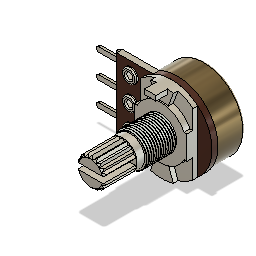
POT10K (Autodesk Fusion 360 design; units mm, degrees)
Autodesk Fusion 360 part; units mm, degrees
sketch "Sketch1" plane through (0, 0, 0) normal (0, 0, 1) x (1, 0, 0)
  circle A0 centre (0, 0) radius 8.2
  dimension "d1" = 16.4
  constraint coincident A0.centre origin
  measures "d1" diameter of A0
extrude "Extrude1" add sketch "Sketch1" along normal blind 6
sketch "Sketch2" plane through (0, 0, 6) normal (0, 0, 1) x (1, 0, 0)
  circle A0 centre (0, 0) radius 8.2
  line L0 (0, 0) -> (-11.5, 0)
  line L1 (-11.5, 0) -> (-11.5, 7.6)
  line L2 (-11.5, 7.6) -> (-3.8066, 7.6)
  line L3 (-11.5, 0) -> (-11.5, -7.6)
  line L4 (-11.5, -7.6) -> (-3.8066, -7.6)
  arc A1 (-3.8066, -7.6) -> (-3.8066, 7.6) centre (0, 0) ccw
  dimension "d4" = 17
  dimension "d5" = 11.5
  dimension "d6" = 7.6
  dimension "d7" = 7.6
  constraint concentric A0 A1
  constraint coincident A0.centre L0.start
  constraint horizontal L0
  constraint perpendicular L0 L1
  constraint perpendicular L1 L2
  constraint perpendicular L0 L3
  constraint perpendicular L3 L4
  measures "d4" diameter of A1
  measures "d5" distance of A0.centre L0.end
  measures "d6" distance of L0.end L1.end
  measures "d7" distance of L0.end L3.end
extrude "Extrude2" add sketch "Sketch2" along normal blind 1.25 contours A0 | L1 L2 L3 L4 A1
fillet "Fillet1" radius 0.5 1 edges at (-7.6451, -2.9652, 0)
sketch "Sketch3" plane through (0, 0, 7.25) normal (0, 0, 1) x (1, 0, 0)
  line L0 (-11.5, 7.6) -> (-11.5, -7.6)
  line L1 (-11.5, -7.6) -> (-3.8066, -7.6)
  arc A0 (-3.8066, -7.6) -> (-3.8066, 7.6) centre (0, 0) ccw
  line L2 (-3.8066, 7.6) -> (-11.5, 7.6)
  circle A1 centre (0, 0) radius 8.5
  line L3 (-5.5, 0) -> (-5.5, 6.4807)
  line L4 (5.5, 6.4807) -> (5.5, -6.4807)
  line L5 (-5.5, -6.4807) -> (-5.5, 0)
  circle A2 centre (0, 0) radius 8.495
  dimension "d15" = 16.99
  constraint concentric A0 A1
  constraint vertical L3
  constraint coincident A1 L3.end
  constraint coincident A0 L4.start
  constraint coincident A1 L5.start
  constraint coincident A0 L4.end
  constraint concentric A1 A2
  measures "d15" diameter of A2
extrude "Extrude3" add sketch "Sketch3" along normal blind 1 contours A0 A1 L3 L4 A2 | A0 A1 L4 L5 A2 | L3 L4 L5 A2
sketch "Sketch4" plane through (0, 0, 8.25) normal (0, 0, 1) x (1, 0, 0)
  arc A0 (-5.5, -6.4742) -> (5.5, -6.4742) centre (0, 0) ccw
  line L0 (5.5, -6.4742) -> (5.5, 6.4742)
  arc A1 (5.5, 6.4742) -> (-5.5, 6.4742) centre (0, 0) ccw
  line L1 (-5.5, 6.4742) -> (-5.5, -6.4742)
  line L2 (5.5, 0) -> (5.5, 2.5)
  line L3 (-5.5, 2.5) -> (-5.5, -2.5)
  line L4 (5.5, -2.5) -> (5.5, 0)
  line L5 (-5.5, -2.5) -> (-4.899, -2.5)
  line L6 (4.899, -2.5) -> (5.5, -2.5)
  arc A2 (-4.899, -2.5) -> (4.899, -2.5) centre (0, 0) ccw
  arc A3 (4.899, 2.5) -> (-4.899, 2.5) centre (0, 0) ccw
  line L7 (5.5, 2.5) -> (4.899, 2.5)
  line L8 (-4.899, 2.5) -> (-5.5, 2.5)
  dimension "d18" = 2.5
  dimension "d19" = 5
  constraint coincident A0.centre A1.centre
  constraint tangent L0 A2
  constraint midpoint L0 L2.start
  constraint parallel L0 L2
  constraint coincident L1 L3.start
  constraint perpendicular L1 L7
  constraint perpendicular L3 L7
  constraint coincident L0 L4.start
  constraint perpendicular L0 L5
  constraint coincident A3.end L7
  constraint collinear L5 L6
  constraint concentric A2 A3
  constraint collinear L7 L8
  measures "d18" distance of L2.start L2.end
  measures "d19" distance of L3.start L3.end
extrude "Extrude4" add sketch "Sketch4" along normal blind 1.25 contours L0 L1 L2 L3 L4 L5 L6 A2 A3 L7 L8
sketch "Sketch5" plane through (0, 0, 8.25) normal (0, 0, 1) x (1, 0, 0)
  line L0 (5.5, -2.5) -> (4.899, -2.5)
  arc A0 (-4.899, -2.5) -> (4.899, -2.5) centre (0, 0) ccw
  line L1 (-4.899, -2.5) -> (-5.5, -2.5)
  line L2 (-5.5, -2.5) -> (-5.5, -6.4742)
  arc A1 (-5.5, -6.4742) -> (5.5, -6.4742) centre (0, 0) ccw
  line L3 (5.5, -6.4742) -> (5.5, -2.5)
  circle A2 centre (0, 0) radius 8.495
  line L4 (0, 0) -> (1.35, 0)
  line L5 (1.35, 0) -> (1.35, 0.0007)
  circle A3 centre (0, 0) radius 5.5
  line L6 (-1.35, 5.3317) -> (-2.4, 8.1489)
  line L7 (1.35, 5.3317) -> (2.4, 8.1489)
  line L8 (1.35, -5.3317) -> (2.4, -8.1489)
  line L9 (-2.3914, -8.1514) -> (-1.35, -5.3317)
  dimension "d23" = 1.35
  dimension "d26" = 11
  constraint coincident A0.centre A1.centre
  constraint horizontal L4
  constraint coincident A2 L7.end
  constraint coincident A2 L6.end
  constraint coincident A1 L9.start
  constraint coincident A2 L9.start
  constraint coincident A1 L8.end
  constraint coincident A3 L6.start
  constraint coincident A3 L7.start
  constraint coincident A3 L8.start
  constraint coincident A3 L9.end
  measures "d23" distance of A0.centre L5.end
  measures "d26" diameter of A3
extrude "Extrude5" add sketch "Sketch5" along normal blind 1 contours A0 A1 A2 A3 L8 L9 | A2 A3 L6 L7
sketch "Sketch6" plane through (0, 0, 9.25) normal (0, 0, 1) x (1, 0, 0)
  arc A0 (1.35, 5.3317) -> (-1.35, 5.3317) centre (0, 0) ccw
  line L0 (1.35, 5.3317) -> (2.4, 8.1489)
  arc A1 (2.4, 8.1489) -> (-2.4, 8.1489) centre (0, 0) ccw
  line L1 (-2.4, 8.1489) -> (-1.35, 5.3317)
  circle A2 centre (0, 0) radius 7.5
  line L2 (0, 0) -> (1.2, 0)
  line L3 (1.2, 0) -> (1.2, 9)
  line L4 (1.2, 9) -> (-1.2, 9)
  line L5 (-1.2, 9) -> (-1.2, 6.8335)
  dimension "d29" = 15
  dimension "d30" = 1.2
  dimension "d31" = 2.4
  constraint concentric A0 A2
  constraint coincident A0.centre A1.centre
  constraint horizontal L2
  constraint perpendicular L2 L3
  constraint perpendicular L3 L4
  constraint perpendicular L4 L5
  measures "d29" diameter of A2
  measures "d30" distance of A0.centre L2.end
  measures "d31" distance of L3.end L4.end
extrude "Extrude6" add sketch "Sketch6" along normal blind 2.5 contours A1 A2 L3 L5
sketch "Sketch7" plane through (0, 0, 9.5) normal (0, 0, 1) x (1, 0, 0)
  line L0 (-4.899, 2.5) -> (-5.5, 2.5)
  line L1 (-5.5, 2.5) -> (-5.5, -2.5)
  line L2 (-5.5, -2.5) -> (-4.899, -2.5)
  arc A0 (-4.899, -2.5) -> (4.899, -2.5) centre (0, 0) ccw
  line L3 (4.899, -2.5) -> (5.5, -2.5)
  line L4 (5.5, -2.5) -> (5.5, 2.5)
  line L5 (5.5, 2.5) -> (4.899, 2.5)
  arc A1 (4.899, 2.5) -> (-4.899, 2.5) centre (0, 0) ccw
  circle A2 centre (0, 0) radius 3.5
  dimension "d34" = 7
  constraint coincident A0.centre A1.centre
  measures "d34" diameter of A2
extrude "Extrude7" add sketch "Sketch7" along normal blind 6.4 contours A2
thread "Thread1" "ISO Metric profile 7.0 M7x0.5 6g" major diameter 6.927 minor diameter 6.3505 pitch 0.5 angle 60 modelled right hand crest width 0.0685 on face at (3.4547, -0.5614, 13.7667) crest through (3.4635, 0, 9.375)
sketch "Sketch8" plane through (0, 0, 15.9) normal (0, 0, 1) x (1, 0, 0)
  spline S0 degree 3 poles (-1.8886, -2.5525) (-1.5648, -2.8146) (-1.1927, -3.0103) (-0.3879, -3.2513) (0.0378, -3.2917) (0.8877, -3.2078) (1.3036, -3.0816) (2.0704, -2.6747) (2.4127, -2.3957) (2.8876, -1.8243) (3.0502, -1.5642) (3.3033, -1.0046) (3.392, -0.7075) (3.44, -0.4025) knots 0 0 0 0 0.124949 0.124949 0.251948 0.251948 0.380996 0.380996 0.512093 0.512093 0.60358 0.60358 0.696049 0.696049 0.696049 0.696049
  arc A0 (3.44, -0.4025) -> (2.5464, 2.3476) centre (0, 0) ccw
  spline S1 degree 3 poles (2.5464, 2.3476) (2.2304, 2.6642) (1.8561, 2.9164) (1.0377, 3.2593) (0.6025, 3.3492) (-0.2709, 3.3556) (-0.7006, 3.2748) (-1.4981, 2.9543) (-1.8591, 2.7203) (-2.3721, 2.2213) (-2.5516, 1.9927) (-2.8429, 1.4963) (-2.9541, 1.2313) (-3.0282, 0.955) knots 0 0 0 0 0.134177 0.134177 0.266302 0.266302 0.396376 0.396376 0.524397 0.524397 0.611348 0.611348 0.697316 0.697316 0.697316 0.697316
  arc A1 (-3.0282, 0.955) -> (-1.8886, -2.5525) centre (0, 0) ccw
  circle A2 centre (0, 0) radius 3.05
  dimension "d37" = 6.1
  constraint concentric A0 A2
  measures "d37" diameter of A2
extrude "Extrude8" add sketch "Sketch8" along normal blind 8.3 contours A2
chamfer "Chamfer1" distance 0.5 angle 45 1 edges at (-2.8436, -1.1029, 24.2)
sketch "Sketch9" plane through (0, 0, 24.2) normal (0, 0, 1) x (1, 0, 0)
  circle A0 centre (0, 0) radius 2.55
  circle A1 centre (0, 0) radius 3.05
  circle A2 centre (0, 0) radius 2.55
  line L0 (0, 0) -> (0, 3.05)
  line L1 (0, 0) -> (1.1557, 3.557)
  line L2 (0, 0) -> (0.3989, 2.5186)
  line L3 (0, 0) -> (2.55, 0) construction
  line L4 (0, 3.05) -> (0.3989, 2.5186)
  line L5 (0.9425, 2.9007) -> (0.3989, 2.5186)
  line L6 (0, 3.05) -> (-0.3989, 2.5186)
  line L7 (-0.9425, 2.9007) -> (-0.3989, 2.5186)
  line L8 (-0.9425, 2.9007) -> (-1.1577, 2.2721)
  line L9 (-1.7927, 2.4675) -> (-1.1577, 2.2721)
  line L10 (-1.7927, 2.4675) -> (-1.8031, 1.8031)
  line L11 (-2.4675, 1.7927) -> (-1.8031, 1.8031)
  line L12 (-2.4675, 1.7927) -> (-2.2721, 1.1577)
  line L13 (-2.9007, 0.9425) -> (-2.2721, 1.1577)
  line L14 (-2.9007, 0.9425) -> (-2.5186, 0.3989)
  line L15 (-3.05, 0) -> (-2.5186, 0.3989)
  line L16 (-3.05, 0) -> (-2.5186, -0.3989)
  line L17 (-2.9007, -0.9425) -> (-2.5186, -0.3989)
  line L18 (-2.9007, -0.9425) -> (-2.2721, -1.1577)
  line L19 (-2.4675, -1.7927) -> (-2.2721, -1.1577)
  line L20 (-2.4675, -1.7927) -> (-1.8031, -1.8031)
  line L21 (-1.7927, -2.4675) -> (-1.8031, -1.8031)
  line L22 (-1.7927, -2.4675) -> (-1.1577, -2.2721)
  line L23 (-0.9425, -2.9007) -> (-1.1577, -2.2721)
  line L24 (-0.9425, -2.9007) -> (-0.3989, -2.5186)
  line L25 (0, -3.05) -> (-0.3989, -2.5186)
  line L26 (0, -3.05) -> (0.3989, -2.5186)
  line L27 (0.9425, -2.9007) -> (0.3989, -2.5186)
  line L28 (0.9425, -2.9007) -> (1.1577, -2.2721)
  line L29 (1.7927, -2.4675) -> (1.1577, -2.2721)
  line L30 (1.7927, -2.4675) -> (1.8031, -1.8031)
  line L31 (2.4675, -1.7927) -> (1.8031, -1.8031)
  line L32 (2.4675, -1.7927) -> (2.2721, -1.1577)
  line L33 (2.9007, -0.9425) -> (2.2721, -1.1577)
  line L34 (2.9007, -0.9425) -> (2.5186, -0.3989)
  line L35 (3.05, 0) -> (2.5186, -0.3989)
  line L36 (3.05, 0) -> (2.5186, 0.3989)
  line L37 (2.9007, 0.9425) -> (2.5186, 0.3989)
  line L38 (2.9007, 0.9425) -> (2.2721, 1.1577)
  line L39 (2.4675, 1.7927) -> (2.2721, 1.1577)
  line L40 (2.4675, 1.7927) -> (1.8031, 1.8031)
  line L41 (1.7927, 2.4675) -> (1.8031, 1.8031)
  line L42 (1.7927, 2.4675) -> (1.1577, 2.2721)
  line L43 (0.9425, 2.9007) -> (1.1577, 2.2721)
  dimension "d41" = 6.1
  dimension "d42" = 162
  dimension "d43" = 81
  dimension "d45" = 360
  constraint concentric A0 A1
  constraint concentric A1 A2
  constraint coincident A0.centre A1.centre
  constraint coincident A1 L0.end
  constraint vertical L0
  constraint horizontal L3
  constraint coincident A2 L2.end
  constraint coincident L1 L5.start
  constraint coincident A1 L5.start
  measures "d41" diameter of A1
  measures "d42" angle of L0 L1
  measures "d43" angle of L2 L3
extrude "Extrude9" cut sketch "Sketch9" against normal blind 6.7 contours A1 L36 L37 | A1 L34 L35 | A1 L38 L39 | A1 L32 L33 | A1 L40 L41 | A1 L30 L31 | A1 L42 L43 | A1 L28 L29 | A1 L4 L5 | A1 L26 L27 | A1 L6 L7 | A1 L24 L25 | A1 L8 L9 | A1 L22 L23 | A1 L10 L11 | A1 L20 L21 | A1 L12 L13 | A1 L18 L19 | A1 L14 L15 | A1 L16 L17
sketch "Sketch10" plane through (0, 0, 24.2) normal (0, 0, 1) x (1, 0, 0)
  arc A0 (-2.5186, 0.3989) -> (-2.5186, -0.3989) centre (0, 0) ccw
  arc A1 (-2.5186, -0.3989) -> (-2.2721, -1.1577) centre (0, 0) ccw
  arc A2 (-2.2721, -1.1577) -> (-1.8031, -1.8031) centre (0, 0) ccw
  arc A3 (-1.8031, -1.8031) -> (-1.1577, -2.2721) centre (0, 0) ccw
  arc A4 (-1.1577, -2.2721) -> (-0.3989, -2.5186) centre (0, 0) ccw
  arc A5 (-0.3989, -2.5186) -> (0.3989, -2.5186) centre (0, 0) ccw
  arc A6 (0.3989, -2.5186) -> (1.1577, -2.2721) centre (0, 0) ccw
  arc A7 (1.1577, -2.2721) -> (1.8031, -1.8031) centre (0, 0) ccw
  arc A8 (1.8031, -1.8031) -> (2.2721, -1.1577) centre (0, 0) ccw
  arc A9 (2.2721, -1.1577) -> (2.5186, -0.3989) centre (0, 0) ccw
  arc A10 (2.5186, -0.3989) -> (2.5186, 0.3989) centre (0, 0) ccw
  arc A11 (2.5186, 0.3989) -> (2.2721, 1.1577) centre (0, 0) ccw
  arc A12 (2.2721, 1.1577) -> (1.8031, 1.8031) centre (0, 0) ccw
  arc A13 (1.8031, 1.8031) -> (1.1577, 2.2721) centre (0, 0) ccw
  arc A14 (1.1577, 2.2721) -> (0.3989, 2.5186) centre (0, 0) ccw
  arc A15 (0.3989, 2.5186) -> (-0.3989, 2.5186) centre (0, 0) ccw
  arc A16 (-0.3989, 2.5186) -> (-1.1577, 2.2721) centre (0, 0) ccw
  arc A17 (-1.1577, 2.2721) -> (-1.8031, 1.8031) centre (0, 0) ccw
  arc A18 (-1.8031, 1.8031) -> (-2.2721, 1.1577) centre (0, 0) ccw
  arc A19 (-2.2721, 1.1577) -> (-2.5186, 0.3989) centre (0, 0) ccw
  line L0 (0, 0) -> (4.1558, 0)
  line L1 (4.1558, 0) -> (4.1558, 0.62)
  line L2 (4.1558, 0.62) -> (-4, 0.62)
  line L3 (-4, 0.62) -> (-4, -0.62)
  line L4 (-4, -0.62) -> (4.1558, -0.62)
  line L5 (4.1558, -0.62) -> (4.1558, 0)
  dimension "d48" = 0.62
  dimension "d49" = 1.24
  constraint coincident A0.centre A1.centre
  constraint horizontal L0
  constraint perpendicular L0 L1
  constraint perpendicular L1 L2
  constraint perpendicular L2 L3
  constraint perpendicular L1 L4
  constraint perpendicular L0 L5
  measures "d48" distance of L0.end L1.end
  measures "d49" distance of L2.end L3.end
extrude "Extrude10" cut sketch "Sketch10" against normal blind 6.7 contours A0 A1 A9 A10 A11 A19 L2 L4 | A0 A1 A19 L2 L3 L4 | A10 A11 L0 L1 L2 | A9 A10 L0 L4 L5
sketch "Sketch11" plane through (0, 0, 6) normal (0, 0, -1) x (-1, 0, 0)
  line L0 (11.5, -7.6) -> (11.5, 7.6)
  line L1 (11.5, 7.6) -> (3.8066, 7.6)
  arc A0 (3.8066, 7.6) -> (3.8066, -7.6) centre (0, 0) ccw
  line L2 (3.8066, -7.6) -> (11.5, -7.6)
  circle A1 centre (0, 0) radius 8.2
  circle A2 centre (0, 0) radius 8.2
  line L3 (0, 0) -> (12.5, 0)
  line L4 (12.5, 0) -> (12.5, 5.2)
  line L5 (12.5, 5.2) -> (6.3403, 5.2)
  line L6 (6.3403, 5.2) -> (6.3403, -5.2)
  dimension "d52" = 5.2
  constraint coincident A0.centre A1.centre
  constraint perpendicular L0 L3
  constraint perpendicular L3 L4
  constraint coincident A2 L5.end
  constraint perpendicular L0 L5
  constraint coincident A1 L6.end
  constraint perpendicular L3 L6
  measures "d52" distance of L3.end L4.end
extrude "Extrude11" cut sketch "Sketch11" along normal blind 2 contours A1 A2 L3 L6 | A1 A2 L3 L6
sketch "Sketch12" plane through (0, 0, 6) normal (0, 0, -1) x (-1, 0, 0)
  line L0 (11.5, -7.6) -> (11.5, 7.6)
  line L1 (11.5, 7.6) -> (3.8066, 7.6)
  arc A0 (3.8066, 7.6) -> (3.8066, -7.6) centre (0, 0) ccw
  line L2 (3.8066, -7.6) -> (11.5, -7.6)
  arc A1 (6.3403, 5.2) -> (6.3403, -5.2) centre (0, 0) ccw
  line L3 (6.3403, 5.2) -> (6.3403, -5.2)
  line L4 (11.5, 0) -> (12.7, 0)
  line L5 (12.7, 0) -> (12.7, -1.75)
  line L6 (12.7, -1.75) -> (8.45, -1.75)
  line L7 (8.45, 1.75) -> (12.7, 1.75)
  line L8 (12.7, 1.75) -> (12.7, 0)
  arc A2 (6.7, 0) -> (8.45, -1.75) centre (8.45, 0) ccw
  arc A3 (8.45, 1.75) -> (6.7, 0) centre (8.45, 0) ccw
  circle A4 centre (8.45, 0) radius 0.65
  line L9 (12.7, 3.33) -> (8.45, 3.33)
  line L10 (12.7, 5.08) -> (12.7, 3.33)
  line L11 (12.7, 6.83) -> (12.7, 5.08)
  line L12 (8.45, 6.83) -> (12.7, 6.83)
  arc A5 (8.45, 6.83) -> (6.7, 5.08) centre (8.45, 5.08) ccw
  arc A6 (6.7, 5.08) -> (8.45, 3.33) centre (8.45, 5.08) ccw
  circle A7 centre (8.45, 5.08) radius 0.65
  line L13 (12.7, -6.83) -> (8.45, -6.83)
  line L14 (12.7, -5.08) -> (12.7, -6.83)
  line L15 (12.7, -3.33) -> (12.7, -5.08)
  line L16 (8.45, -3.33) -> (12.7, -3.33)
  arc A8 (8.45, -3.33) -> (6.7, -5.08) centre (8.45, -5.08) ccw
  arc A9 (6.7, -5.08) -> (8.45, -6.83) centre (8.45, -5.08) ccw
  circle A10 centre (8.45, -5.08) radius 0.65
  point P0 (6.7, -1.75)
  point P1 (6.7, 1.75)
  dimension "d55" = 1.2
  dimension "d56" = 1.75
  dimension "d57" = 6
  dimension "d58" = 3.5
  dimension "d59" = 1.75
  dimension "d60" = 1.75
  dimension "d61" = 1.3
  dimension "d64" = 0
  dimension "d65" = -5.08
  constraint midpoint L0 L4.start
  constraint perpendicular L0 L4
  constraint perpendicular L4 L5
  constraint perpendicular L5 L6
  constraint perpendicular L5 L7
  constraint perpendicular L4 L8
  constraint coincident P0 L6
  constraint tangent L6 A2
  constraint coincident P1 L7
  constraint tangent L7 A3
  constraint coincident A2.start A3.end
  constraint concentric A3 A4
  measures "d55" distance of L4.start L4.end
  measures "d56" distance of L4.end L5.end
  measures "d57" distance of L5.end P0
  measures "d58" distance of P0 P1
  measures "d59" radius of A2
  measures "d60" radius of A3
  measures "d61" diameter of A4
extrude "Extrude12" add sketch "Sketch12" along normal blind 0.5 contours L0 L13 L16 A8 A9 | L0 L13 L14 L15 L16 | L0 L6 L7 A2 A3 | L0 L4 L5 L6 | L0 L4 L7 L8 | L0 L9 L10 L11 L12 | L0 L9 L12 A5 A6
extrude "Extrude13" cut 1 faces at (-8.3708, -5.2817, 6) along direction (0, 0, 1) blind 1.25
extrude "Extrude14" cut 1 faces at (-8.271, -0.1221, 6) along direction (0, 0, 1) blind 4
extrude "Extrude15" cut 1 faces at (-8.3708, 4.8783, 6) along direction (0, 0, 1) blind 5
sketch "Sketch13" plane through (0, 0, 7.25) normal (0, 0, 1) x (1, 0, 0)
  circle A0 centre (-8.45, 5.08) radius 0.65
  circle A1 centre (-8.45, 0) radius 0.65
  circle A2 centre (-8.45, -5.08) radius 0.65
  line L0 (-5.5, -6.4742) -> (-5.5, 6.4742)
  arc A3 (5.5, 6.4742) -> (-5.5, 6.4742) centre (0, 0) ccw
  line L1 (5.5, 6.4742) -> (5.5, -6.4742)
  arc A4 (-5.5, -6.4742) -> (5.5, -6.4742) centre (0, 0) ccw
  line L2 (-11.5, 7.6) -> (-11.5, -7.6)
  line L3 (-11.5, -7.6) -> (-3.8066, -7.6)
  arc A5 (-3.8066, -7.6) -> (-3.8066, 7.6) centre (0, 0) ccw
  line L4 (-3.8066, 7.6) -> (-11.5, 7.6)
  circle A6 centre (-8.45, -5.08) radius 1.5
  circle A7 centre (-8.45, 0) radius 1.5
  circle A8 centre (-8.45, 5.08) radius 1.5
  dimension "d74" = 3
  dimension "d75" = 3
  dimension "d76" = 3
  constraint concentric A2 A6
  constraint concentric A1 A7
  constraint concentric A0 A8
  measures "d74" diameter of A6
  measures "d75" diameter of A7
  measures "d76" diameter of A8
extrude "Extrude16" add sketch "Sketch13" along normal blind 0.5 contours A6 | A7 | A8
fillet "Fillet2" radius 0.25 6 edges at (-9.056, 5.3151, 7.75) (-9.8485, 4.5376, 7.75) (-9.8485, -0.5424, 7.75) (-9.056, 0.2351, 7.75) (-9.8485, -5.6224, 7.75) (-9.056, -4.8449, 7.75)
sketch "Sketch15" plane through (-12.7, 0, 0) normal (-1, 0, 0) x (0, 0, 1)
  line L0 (6, -1.75) -> (6, 1.75)
  line L1 (6, 1.75) -> (5.5, 1.75)
  line L2 (5.5, 1.75) -> (5.5, -1.75)
  line L3 (5.5, -1.75) -> (6, -1.75)
  line L4 (6, 0) -> (6, -0.5)
  line L5 (6, -0.5) -> (5.5, -0.5)
  line L6 (5.5, -0.5) -> (5.5, 0.5)
  line L7 (5.5, 0.5) -> (6, 0.5)
  line L8 (6, 0.5) -> (6, 0)
  line L9 (6, 0) -> (6, -5.08)
  line L10 (6, -5.08) -> (6, -5.58)
  line L11 (6, -5.58) -> (5.5, -5.58)
  line L12 (5.5, -5.58) -> (5.5, -4.58)
  line L13 (5.5, -4.58) -> (6, -4.58)
  line L14 (6, -4.58) -> (6, -5.58)
  line L15 (6, 0) -> (6, 5.08)
  line L16 (6, 5.08) -> (6, 5.58)
  line L17 (6, 5.58) -> (5.5, 5.58)
  line L18 (5.5, 5.58) -> (5.5, 4.58)
  line L19 (5.5, 4.58) -> (6, 4.58)
  line L20 (6, 4.58) -> (6, 5.08)
  dimension "d94" = 0.5
  dimension "d95" = 5.08
  dimension "d96" = 0.5
  dimension "d97" = 1
  dimension "d98" = 5.08
  dimension "d99" = 0.5
  dimension "d100" = 1
  constraint midpoint L0 L4.start
  constraint parallel L0 L4
  constraint coincident L2 L5.end
  constraint perpendicular L2 L5
  constraint coincident L2 L6.end
  constraint coincident L0 L7.end
  constraint perpendicular L0 L7
  constraint perpendicular L3 L9
  constraint parallel L9 L10
  constraint perpendicular L10 L11
  constraint perpendicular L11 L12
  constraint coincident L9 L13.end
  constraint perpendicular L9 L13
  constraint parallel L0 L15
  constraint parallel L15 L16
  constraint perpendicular L16 L17
  constraint perpendicular L17 L18
  constraint coincident L15 L19.end
  constraint perpendicular L15 L19
  measures "d94" distance of L4.start L4.end
  measures "d95" distance of L4.start L9.end
  measures "d96" distance of L9.end L10.end
  measures "d97" distance of L11.end L12.end
  measures "d98" distance of L4.start L15.end
  measures "d99" distance of L15.end L16.end
  measures "d100" distance of L17.end L18.end
extrude "Extrude18" add sketch "Sketch15" along normal blind 4.3 contours L0 L2 L4 L5 L6 L7 L8 L9 L15 | L9 L10 L11 L12 L13 L14 | L15 L16 L17 L18 L19 L20
fillet "Fillet5" radius 0.5 3 edges at (-17, -4.58, 5.75) (-17, 0.5, 5.75) (-17, 5.58, 5.75)
fillet "Fillet6" radius 0.5 3 edges at (-17, -5.58, 5.75) (-17, -0.5, 5.75) (-17, 4.58, 5.75)
equation "d6 = ( 15.2 / 2 ) * 1 mm"
equation "d48 = ( 1.24 / 2 ) * 1 mm"
equation "d56 = ( 3.5 / 2 ) * 1 mm"
